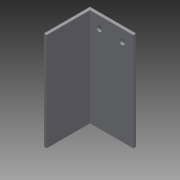
# Autodesk Inventor part: 2x2 angle vertical left
Saved by Autodesk Inventor 2015 SP1 (Build 190203100, 203)
## iProperties
Created: 2015-01-16
Part Number: 2x2 angle vertical left
Material: Generic
Document SubType Name: Modeling
Designer: Jarod
Density: 1 g/cm^3
Appearance: Default
Author: Jarod
Autodesk Inventor part; units mm, degrees
ref_plane "YZ Plane" through (0, 0, 0) normal (1, 0, 0) x (0, 1, 0)
ref_plane "XZ Plane" through (0, 0, 0) normal (0, 1, 0) x (-1, 0, 0)
ref_plane "XY Plane" through (0, 0, 0) normal (0, 0, 1) x (1, 0, 0)
sketch "Sketch1" plane through (0, 0, 0) normal (0, 1, 0) x (-1, 0, 0)
  line L0 (0, 0) -> (-3.175, 0)
  line L1 (-3.175, 0) -> (-3.175, 50.8)
  line L2 (-3.175, 50.8) -> (0, 50.8)
  line L3 (0, 50.8) -> (0, 0)
  line L4 (0, 0) -> (-50.8, 0)
  line L5 (-50.8, 0) -> (-50.8, 3.175)
  line L6 (-50.8, 3.175) -> (0, 3.175)
  line L7 (0, 3.175) -> (0, 0)
  dimension "d0" = 3.175
  dimension "d1" = 50.8
  dimension "d2" = 50.8
  dimension "d3" = 3.175
  constraints: 16 end point, 4 parallel, 2 horizontal, 2 perpendicular
  measures "d0" distance of L1.end L2.end
  measures "d1" distance of L0.end L1.end
  measures "d2" distance of L5.end L6.end
  measures "d3" distance of L4.end L5.end
extrude "Extrusion1" add sketch "Sketch1" against normal blind 139.7
sketch "Sketch2" plane through (50.8, 0, 0) normal (0, 0, -1) x (-1, 0, 0)
  line L0 (50.8, -139.7) -> (0, -139.7) projected
  line L1 (50.8, 0) -> (50.8, -139.7) projected
  line L2 (0, 0) -> (50.8, 0) projected
  line L3 (0, 0) -> (0, -139.7) projected
  point P0 (12.7, -12.7)
  point P1 (38.1, -12.7)
  dimension "d6" = 12.7
  dimension "d7" = 12.7
  dimension "d8" = 12.7
  dimension "d9" = 12.7
  measures "d6" distance from line of point (38.1, -12.7) L1
  measures "d7" distance from line of L3 point (12.7, -12.7)
  measures "d8" distance from line of L2 point (12.7, -12.7)
  measures "d9" distance from line of L2 point (38.1, -12.7)
hole "Hole1" at (38.1, -12.7, 0) at (12.7, -12.7, 0) direction (0, 0, 1) diameter 6.35 end through all
sketch "Sketch3" plane through (0, 0, 0) normal (-1, 0, 0) x (0, 0, 1)
  line L0 (0, 0) -> (50.8, 0) projected
  line L1 (0, 0) -> (0, -139.7) projected
  line L2 (50.8, -139.7) -> (0, -139.7) projected
  line L3 (50.8, 0) -> (50.8, -139.7) projected
  point P0 (15.875, -127)
  point P1 (41.275, -127)
  dimension "d17" = 9.525
  dimension "d18" = 12.7
  dimension "d19" = 12.7
  dimension "d20" = 15.875
  measures "d17" distance from line of L3 point (41.275, -127)
  measures "d18" distance from line of L2 point (41.275, -127)
  measures "d19" distance from line of L2 point (15.875, -127)
  measures "d20" distance from line of L1 point (15.875, -127)
hole "Hole2" at (0, -127, 15.875) at (0, -127, 41.275) direction (1, 0, 0) diameter 6.35 end through all
sketch "Sketch4" plane through (50.8, 0, 0) normal (0, 0, -1) x (-1, 0, 0)
  circle A0 centre (12.7, -12.7) radius 3.175 projected
  circle A1 centre (38.1, -12.7) radius 3.175 projected
  line L0 (50.8, -139.7) -> (0, -139.7) projected
  line L1 (50.8, 0) -> (50.8, -139.7) projected
  line L2 (0, 0) -> (50.8, 0) projected
  line L3 (0, 0) -> (0, -139.7) projected
  point P0 (22.225, -50.8)
  point P1 (22.225, -88.9)
  dimension "d28" = 28.575
  dimension "d29" = 28.575
  dimension "d30" = 50.8
  dimension "d31" = 88.9
  measures "d28" distance from line of point (22.225, -50.8) L1
  measures "d29" distance from line of L1 point (22.225, -88.9)
  measures "d30" distance from line of L2 point (22.225, -50.8)
  measures "d31" distance from line of point (22.225, -88.9) L2
hole "Hole3" at (28.575, -50.8, 0) at (28.575, -88.9, 0) direction (0, 0, 1) diameter 6.35 end through all
body "Solid1"
